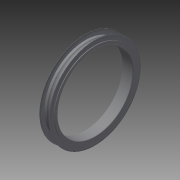
# Autodesk Inventor part: 61814-2RS1_PART1
Saved by Autodesk Inventor 2014 SP2 (Build 180246200, 246)
## iProperties
Created: 2019-11-07
Part Number: 61814-2RS1_PART1
Material: Generic
Catalog Web Link: www.cadenas.de
Description: -Deep groove ball bearings
Vendor: SKF
Document SubType Name: Modeling
Designer: psadmin
Manufacturer: SKF
Mass: 7.26292 g
Surface Area: 106.899 cm^2
Volume: 7.26292 cm^3
Density: 1 g/cm^3
Appearance: PSOLRGB-175-175-175
Category: PARTsolutions
Company: SKF
Title: 61814-2RS1_PART1
Author: Cadenas PARTsolutions
Comments: Deep groove ball bearings
PSOL_IDENT_0: {$CADENAS_DATA\23d-libs\skf\bearings_units_and_housings\ball_bearings\deep_groove_ball_bearings\bb1_
PSOL_IDENT_1: 001_101.prj},198 {VTYP=3D},{NB=61814-2RS1_PART1},{LINA=61814-2RS1_PART1},{NN=BB1_001_101_PART1},{NOP
PSOL_IDENT_2: RJ=TRUE},{DATE=07.11.2019 10:38:24},{GEOMDATE=11.06.2019 11:24:58},{VERSION=},{LINEID=8240},{WBVAR=}
PSOL_IDENT_3: ,{WBNUMERIC=}  {NB=61814-2RS1_PART1},{LINA=61814-2RS1_PART1},{KT=DUMMY},{PRODUCTID=1010271814},{DESI
PSOL_IDENT_4: GNATION=61814-2RS1},{DD=70.00},{D=90.000},{B=10.000},{C=0.000},{DD1=76.40},{DD2=0.0},{D1=0.00},{D2=8
PSOL_IDENT_5: 5.50},{D3=0.00},{D4=0.000},{HH=MIN},{BB=0.000},{FF=0.00},{R0MAX=MIN},{R0=MIN},{R12=0.60},{PITCH=80.0
PSOL_IDENT_6: 0},{DW=5.556},{DDAMIN=73.200},{DDAMAX=76.500},{DDBMIN=MIN},{DDBMAX=MIN},{DBMIN=MIN},{DAMAX=86.800},{
PSOL_IDENT_7: BBAMIN=MIN},{CAMAX=MIN},{RAMAX=0.600},{LOAD1=12.400},{LOAD2=13.200},{LOAD3=0.560},{SPEED1=MIN},{SPEE
PSOL_IDENT_8: D2=4300},{KR=0.015},{F0=17.200},{Z=24},{II=1},{MASS=0.140},{BEARING=61814-2RS1},{RING=},{HELP=3.139}
PSOL_IDENT_9: ,{HELP2=2.250},{DD1ALG=38.200},{YALG=38.200},{PITCH1=80.000},{DW1=5.556},{YALG1=41.861},{HALG1=3.139
PSOL_IDENT_10: },{SH=38.200},{CU=0.889},{DESIGN=dgbb2rs},{HALG=3.2},{B1=0},{ALGO=1.000}
NT: Deep groove ball bearings
NB: 61814-2RS1_PART1
NBSYN: $DESIGNATION._PART1
LINA: 61814-2RS1_PART1
SUPPLIER: SKF
ARTICLENO: 61814-2RS1_PART1
BOMINFO: 61814-2RS1_PART1
CREATOR: CADENAS GmbH
Autodesk Inventor part; units mm, degrees
ref_plane "YZ Plane" through (0, 0, 0) normal (1, 0, 0) x (0, 1, 0)
ref_plane "XZ Plane" through (0, 0, 0) normal (0, 1, 0) x (-1, 0, 0)
ref_plane "XY Plane" through (0, 0, 0) normal (0, 0, 1) x (1, 0, 0)
sketch "Sketch_58" plane through (0, 0, 0) normal (0, 0, 1) x (1, 0, 0)
  line L0 (50, 0) -> (-50, 0)
  line L1 (0, 38) -> (0, 35.6)
  arc A0 (0, 35.6) -> (0.6, 35) centre (0.6, 35.6) ccw
  line L2 (0.6, 35) -> (9.4, 35)
  arc A1 (9.4, 35) -> (10, 35.6) centre (9.4, 35.6) ccw
  line L3 (10, 35.6) -> (10, 38)
  arc A2 (10, 38) -> (9.8, 38.2) centre (9.8, 38) ccw
  line L4 (9.8, 38.2) -> (7.116, 38.2)
  arc A3 (2.884, 38.2) -> (7.116, 38.2) centre (5, 40) ccw
  line L5 (2.884, 38.2) -> (0.2, 38.2)
  arc A4 (0.2, 38.2) -> (0, 38) centre (0.2, 38) ccw
  constraints: 12 end point, 10 point on circle, 5 centre point
revolve "Revolution1" add sketch "Sketch_58" angle 360 about axis through (50, 0, 0) along (1, 0, 0)
sketch "Sketch_60" plane through (0, 0, 0) normal (0, 0, 1) x (1, 0, 0)
  line L0 (50, 0) -> (-50, 0)
  line L1 (0.54, 42.75) -> (0.63, 41.6125)
  line L2 (0.63, 41.6125) -> (0.54, 40.475)
  line L3 (0.54, 40.475) -> (0.54, 38.2)
  line L4 (0.54, 38.2) -> (0.72, 38.2)
  line L5 (0.72, 38.2) -> (0.9, 40.475)
  line L6 (0.9, 40.475) -> (0.9, 41.6125)
  line L7 (0.9, 41.6125) -> (0.72, 42.75)
  line L8 (0.72, 42.75) -> (0.54, 42.75)
  constraints: 18 end point
revolve "Revolution2" add sketch "Sketch_60" angle 360 about axis through (50, 0, 0) along (1, 0, 0)
sketch "Sketch_61" plane through (0, 0, 0) normal (0, 0, 1) x (1, 0, 0)
  line L0 (50, 0) -> (-50, 0)
  line L1 (9.1, 40.475) -> (9.28, 38.2)
  line L2 (9.28, 38.2) -> (9.46, 38.2)
  line L3 (9.46, 38.2) -> (9.46, 40.475)
  line L4 (9.46, 40.475) -> (9.37, 41.6125)
  line L5 (9.37, 41.6125) -> (9.46, 42.75)
  line L6 (9.46, 42.75) -> (9.28, 42.75)
  line L7 (9.28, 42.75) -> (9.1, 41.6125)
  line L8 (9.1, 41.6125) -> (9.1, 40.475)
  constraints: 18 end point
revolve "Revolution3" add sketch "Sketch_61" angle 360 about axis through (50, 0, 0) along (1, 0, 0)
body "Solid1"
